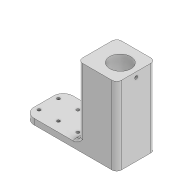
# Autodesk Inventor part: Shaft_Mount_Lower
Saved by Autodesk Inventor 2022 (Build 260153000, 153)
## iProperties
Created: 2022-11-13
Part Number: Shaft_Mount_Lower
Material: Generic
Document SubType Name: Modeling
Designer: MVeszpremi
Density: 1 g/cm^3
Appearance: Default
Author: MVeszpremi
Autodesk Inventor part; units mm, degrees
ref_plane "YZ Plane" through (0, 0, 0) normal (1, 0, 0) x (0, 1, 0)
ref_plane "XZ Plane" through (0, 0, 0) normal (0, 1, 0) x (-1, 0, 0)
ref_plane "XY Plane" through (0, 0, 0) normal (0, 0, 1) x (1, 0, 0)
sketch "Sketch1" plane through (0, 0, 0) normal (0, 1, 0) x (-1, 0, 0)
  line L0 (-20, 10) -> (20, 10)
  line L1 (20, 10) -> (20, -10)
  line L2 (20, -10) -> (-20, -10)
  line L3 (-20, -10) -> (-20, 10)
  line L4 (-20, 10) -> (20, -10) construction
  line L5 (20, 10) -> (-20, -10) construction
  line L6 (-25, 20) -> (25, 20)
  line L7 (25, 20) -> (25, -20)
  line L8 (25, -20) -> (-25, -20)
  line L9 (-25, -20) -> (-25, 20)
  line L10 (-25, 20) -> (25, -20) construction
  line L11 (25, 20) -> (-25, -20) construction
  circle A0 centre (20, 10) radius 1.5
  circle A1 centre (20, -10) radius 1.5
  circle A2 centre (-20, -10) radius 1.5
  circle A3 centre (-20, 10) radius 1.5
  circle A4 centre (0, -10) radius 1.5
  circle A5 centre (0, 10) radius 1.5
  point P0 (0, 0)
  dimension "d0" = 40
  dimension "d1" = 20
  dimension "d2" = 50
  dimension "d3" = 40
  dimension "d4" = 3
  dimension "d5" = 3
  dimension "d6" = 3
  dimension "d7" = 3
  dimension "d31" = 3
  dimension "d32" = 3
  constraints: 24 end point, 6 centre point, 6 midpoint, 4 coincident, 4 parallel, 2 horizontal, 2 perpendicular
  measures "d0" distance of L0.start L0.end
  measures "d1" distance of L0.end L1.end
  measures "d2" distance of L7.end L8.end
  measures "d3" distance of L6.end L7.end
  measures "d4" diameter of A0
  measures "d5" diameter of A1
  measures "d6" diameter of A3
  measures "d7" diameter of A2
  measures "d31" diameter of A4
  measures "d32" diameter of A5
extrude "Extrusion1" add sketch "Sketch1" along normal blind 6 contours L0 A5 A0 L1 A1 L2 A4 A2 L3 A3 | L6 L7 L8 L9
sketch "Sketch2" plane through (0, 6, 0) normal (0, 1, 0) x (1, 0, 0)
  line L0 (-25, -20) -> (25, -20) projected
  line L1 (25, -20) -> (45, -20)
  line L2 (45, -20) -> (45, 20)
  line L3 (45, 20) -> (25, 20)
  line L4 (25, 20) -> (25, -20)
  point P0 (0, 0)
  dimension "d10" = 20
  constraints: 8 end point, 2 parallel, 1 coincident, 1 horizontal, 1 perpendicular
  measures "d10" distance of L2.end L3.end
extrude "Extrusion2" add sketch "Sketch2" against normal blind 6
sketch "Sketch3" plane through (-25, 0, 20) normal (0, 0, 1) x (1, 0, 0)
  line L0 (70, 0) -> (0, 0) projected
  line L1 (55, 0) -> (95, 0)
  line L2 (95, 0) -> (95, 80)
  line L3 (95, 80) -> (55, 80)
  line L4 (55, 80) -> (55, 0)
  line L5 (70, 6) -> (70, 0) projected
  point P0 (25, 0)
  point P1 (75, 80)
  point P2 (70, 0)
  dimension "d13" = 15
  dimension "d14" = 40
  dimension "d15" = 80
  constraints: 8 end point, 2 parallel, 1 horizontal, 1 midpoint, 1 perpendicular, 1 point on line
  measures "d13" distance between parallel lines of L5 L4
  measures "d14" distance of L2.end L3.end
  measures "d15" distance of L1.end L2.end
extrude "Extrusion3" add sketch "Sketch3" against normal up to surface (40 mm away)
ref_plane "Work Plane1" through (70, 80, 20) normal (0.1650476, 0.9862856, 0) x (0, 0, -1)
sketch "Sketch4" plane through (70, 80, 20) normal (0.1650476, 0.9862856, 0) x (0, 0, -1)
  line L0 (0, 0) -> (40, 0) projected
  line L1 (20, 0) -> (20, 16)
  circle A0 centre (20, 16) radius 10.8
  point P0 (20, 55.8362)
  dimension "d20" = 21.6
  dimension "d21" = 16
  constraints: 2 end point, 1 centre point, 1 coincident, 1 midpoint, 1 vertical
  measures "d20" diameter of A0
  measures "d21" distance of L1.start L1.end
extrude "Extrusion4" cut sketch "Sketch4" against normal blind 50
sketch "Sketch5" plane through (70, 0, 20) normal (1, 0, 0) x (0, 0, -1)
  line L0 (0, 80) -> (40, 80) projected
  line L1 (20, 80) -> (20, 75)
  line L2 (20, 78.4641) -> (23, 76.7321)
  line L3 (23, 76.7321) -> (23, 73.2679)
  line L4 (23, 73.2679) -> (20, 71.5359)
  line L5 (20, 71.5359) -> (17, 73.2679)
  line L6 (17, 73.2679) -> (17, 76.7321)
  line L7 (17, 76.7321) -> (20, 78.4641)
  circle A0 centre (20, 75) radius 1.5
  point P0 (20, 0)
  dimension "d24" = 5
  dimension "d25" = 6
  dimension "d26" = 3
  constraints: 14 end point, 2 coincident, 1 centre point, 1 midpoint, 1 point on line, 1 vertical, 13 other
  measures "d24" distance of L1.start L1.end
  measures "d25" distance between parallel lines of L3 L6
  measures "d26" diameter of A0
extrude "Extrusion5" cut sketch "Sketch5" against normal blind 14.75 contours L2 L3 L4 L5 L6 L7 | A0
extrude "Extrusion6" add sketch "Sketch5" against normal blind 3
fillet "Fillet1" radius 5 4 edges at (30, 43, 20) (70, 40, 20) (30, 43, -20) (70, 40, -20)
fillet "Fillet2" radius 10 2 edges at (-25, 3, -20) (-25, 3, 20)
fillet "Fillet3" radius 6 3 edges at (31.4645, 6, -18.5355) (31.4645, 6, 18.5355) (30, 6, 0)
body "Solid1"
